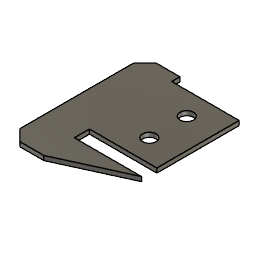
GPL H200 to H150G4 (Autodesk Fusion 360 design; units mm, degrees)
Autodesk Fusion 360 part; units mm, degrees
sketch "スケッチ1" plane through (0, 0, 0) normal (0, 0, 1) x (1, 0, 0)
  line L0 (-21.5, 91) -> (-68.5, 91)
  line L1 (-68.5, 91) -> (-68.5, -91)
  line L2 (-68.5, -91) -> (-21.5, -91)
  line L3 (68.5, -30) -> (68.5, 80)
  line L4 (60.2198, 80) -> (-68.5, -91) construction
  line L5 (-68.5, 91) -> (45.5182, -60.4695) construction
  line L6 (-21.5, 91) -> (-21.5, 80)
  line L7 (-21.5, 80) -> (68.5, 80)
  line L8 (-68.5, -91) -> (-21.5, -91) construction
  line L9 (68.5, -50) -> (-21.5, -91)
  line L10 (68.5, -50) -> (-21.5, -50)
  line L11 (-21.5, -50) -> (-21.5, -30)
  line L12 (-21.5, -30) -> (68.5, -30)
  dimension "d2" = 182
  dimension "d5" = 47
  dimension "d7" = 90
  dimension "d8" = 20
  constraint horizontal L0
  constraint perpendicular L0 L1
  constraint parallel L0 L2
  constraint parallel L1 L3
  constraint coincident L4 origin
  constraint coincident L5 origin
  constraint vertical L6
  constraint horizontal L7
  constraint coincident L7 L4.start
  constraint perpendicular L1 L8
  constraint coincident L9 L5.end
  constraint horizontal L10
  constraint vertical L11
  constraint horizontal L12
  measures "d2" distance of L0.end L1.end
  measures "d5" distance of L1.end L2.end
  measures "d7" distance of L9.start L10.end
  measures "d8" distance of L9.start L3.start
extrude "押し出し1" add sketch "スケッチ1" along normal blind 6
chamfer "面取り1" distance 15 angle 45 2 edges at (-68.5, -91, 3) (-68.5, 91, 3)
sketch "スケッチ2" plane through (0, 0, 6) normal (0, 0, 1) x (-1, 0, 0)
  line L0 (53.5, -91) -> (68.5, -76)
  line L1 (68.5, -76) -> (68.5, 76)
  line L2 (68.5, 76) -> (53.5, 91)
  line L3 (53.5, 91) -> (21.5, 91)
  line L4 (21.5, 91) -> (-68.5, 50)
  line L5 (-68.5, 50) -> (21.5, 50)
  line L6 (21.5, 50) -> (21.5, 30)
  line L7 (21.5, 30) -> (-68.5, 30)
  line L8 (-68.5, 30) -> (-68.5, -80)
  line L9 (-68.5, -80) -> (21.5, -80)
  line L10 (21.5, -80) -> (21.5, -91)
  line L11 (21.5, -91) -> (53.5, -91)
  line L12 (-68.5, -80) -> (-28.5, -80) construction
  line L13 (-28.5, -80) -> (-28.5, -50) construction
  line L14 (-28.5, -50) -> (-68.5, -50) construction
  line L15 (-68.5, -50) -> (-68.5, -80) construction
  line L16 (-28.5, -50) -> (-28.5, 0) construction
  point P0 (-28.5, -50)
  point P1 (-28.5, 0)
  dimension "d12" = 40
  dimension "d13" = 30
  dimension "d14" = 50
  constraint horizontal L12
  constraint vertical L13
  constraint horizontal L14
  constraint vertical L15
  constraint coincident L8.end L9.start
  constraint perpendicular L14 L16
  constraint coincident P0 L13.end
  constraint coincident P1 L16.end
  measures "d12" distance of L8.end L12.end
  measures "d13" distance of L8.end L14.end
  measures "d14" distance of P0 P1
hole "穴1" at (28.5, 0, 6) at (28.5, 50, 6) direction (0, 0, -1) diameter 18 end through all
equation "d5 = 15 mm + 32 mm"
